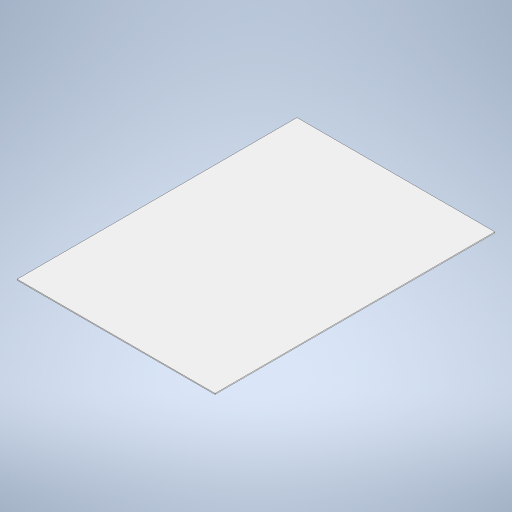
# Autodesk Inventor part: A4
Saved by Autodesk Inventor 2023 (Build 270158000, 158)
## iProperties
Created: 2022-10-06
Part Number: A4
Material: Generic
Document SubType Name: Modeling
Designer: VoorL
Density: 1 g/cm^3
Appearance: White
Author: VoorL
Autodesk Inventor part; units mm, degrees
ref_plane "YZ Plane" through (0, 0, 0) normal (1, 0, 0) x (0, 1, 0)
ref_plane "XZ Plane" through (0, 0, 0) normal (0, 1, 0) x (-1, 0, 0)
ref_plane "XY Plane" through (0, 0, 0) normal (0, 0, 1) x (1, 0, 0)
sketch "Sketch1" plane through (0, 0, 0) normal (0, 1, 0) x (-1, 0, 0)
  line L0 (-105, 148.5) -> (105, 148.5)
  line L1 (105, 148.5) -> (105, -148.5)
  line L2 (105, -148.5) -> (-105, -148.5)
  line L3 (-105, -148.5) -> (-105, 148.5)
  line L4 (-105, 148.5) -> (105, -148.5) construction
  line L5 (105, 148.5) -> (-105, -148.5) construction
  point P0 (0, 0)
  dimension "d0" = 210
  dimension "d1" = 297
  constraints: 12 end point, 2 midpoint, 2 parallel, 1 horizontal, 1 perpendicular
  measures "d0" distance of L1.end L2.end
  measures "d1" distance of L0.end L1.end
extrude "Extrusion1" add sketch "Sketch1" along normal blind 1
body "Solid1"
